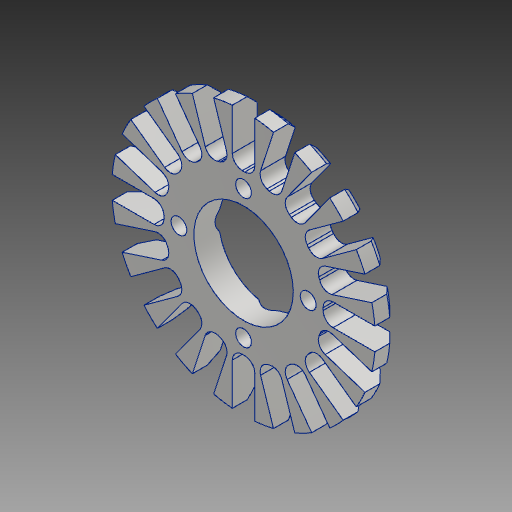
# Autodesk Inventor part: Raddeckel
Saved by Autodesk Inventor 2019.4 (Build 234330000, 330)
## iProperties
Part Number: Raddeckel
Material: Aluminium 6061
Document SubType Name: Modeling
Designer: rYan
Mass: 12.1113 g
Surface Area: 49.3887 cm^2
Volume: 4.48568 cm^3
Density: 2.7 g/cm^3
Appearance: Aluminium - flach
Author: rYan
Autodesk Inventor part; units mm, degrees
ref_plane "YZ Plane" through (0, 0, 0) normal (1, 0, 0) x (0, 1, 0)
ref_plane "XZ Plane" through (0, 0, 0) normal (0, 1, 0) x (-1, 0, 0)
ref_plane "XY Plane" through (0, 0, 0) normal (0, 0, 1) x (1, 0, 0)
sketch "Skizze1" plane through (0, 0, 0) normal (0, 0, 1) x (1, 0, 0)
  line L0 (0, 0) -> (0, 4)
  line L1 (10, 5) -> (24.5, 5)
  line L2 (24.5, 5) -> (26.5, 3)
  line L3 (26.5, 3) -> (26.5, 0)
  line L4 (26.5, 0) -> (10, 0)
  line L5 (10, 0) -> (10, 5)
  dimension "d0" = 5
  dimension "d1" = 20
  dimension "d2" = 53
  dimension "d3" = 45
  dimension "d4" = 3
  constraints: 12 end point, 3 perpendicular, 1 horizontal, 1 point on line, 1 vertical
  measures "d0" distance of L4.end L1.start
  measures "d1" diameter of L5 L0
  measures "d2" diameter of L3 L0
  measures "d3" angle of L2 L3
  measures "d4" distance of L2.end L3.end
revolve "Umdrehung1" add sketch "Skizze1" angle 360 about axis through (0, 0, 0) along (0, 1, 0)
sketch "Skizze2" plane through (0, 0, 0) normal (0, 1, 0) x (-1, 0, 0)
  circle A0 centre (0, 0) radius 16 construction
  circle A1 centre (0, 0) radius 26.5 projected
  line L0 (0, 0) -> (0, 26.5) construction
  line L1 (2.25, 26.5) -> (-2.25, 26.5)
  line L2 (-2.25, 26.5) -> (-2.25, 18)
  line L3 (-0.25, 16) -> (0.25, 16)
  line L4 (2.25, 18) -> (2.25, 26.5)
  arc A2 (0.25, 16) -> (2.25, 18) centre (0.25, 18) ccw
  arc A3 (-2.25, 18) -> (-0.25, 16) centre (-0.25, 18) ccw
  point P0 (-2.25, 16)
  point P1 (2.25, 16)
  dimension "d6" = 32
  dimension "d7" = 4.5
  dimension "d8" = 2
  constraints: 10 end point, 5 tangent, 4 point on circle, 4 point on line, 3 centre point, 2 parallel, 1 coincident, 1 equal radius, 1 horizontal, 1 midpoint, 1 perpendicular, 1 vertical, 1 vertical alignment, 2 other
  measures "d6" diameter of A0
  measures "d7" distance of point (-2.25, 16) point (2.25, 16)
  measures "d8" radius of A2
extrude "Extrusion1" cut sketch "Skizze2" along normal through all contours L4 A2 L3 A3 L2 A1 | A1 L1 L4 | L2 L1 A1 picked at (0, 20.8333)
pattern_circular "Runde Anordnung1" count 20 over 360 about axis through (0, -10, 0) along (0, 1, 0) of "Extrusion1"
sketch "Skizze3" plane through (-2.25, 5, 24.3965) normal (0, 1, 0) x (1, 0, 0)
  circle A0 centre (2.25, 24.3965) radius 13 construction
  line L0 (2.25, 37.3965) -> (2.25, 11.3965) construction
  line L1 (-10.75, 24.3965) -> (15.25, 24.3965) construction
  dimension "d14" = 26
  constraints: 5 coincident, 4 end point, 4 point on circle, 3 midpoint, 1 centre point, 1 perpendicular, 1 vertical
  measures "d14" diameter of A0
hole "Bohrung1" at (-13, 5, 0) at (0, 5, -13) at (13, 5, 0) at (0, 5, 13) direction (0, -1, 0) diameter 3.2 end through all countersink diameter 7.5 countersink angle 90
